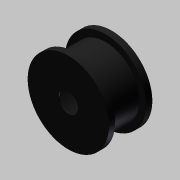
# Autodesk Inventor part: MSK01-06
Saved by Autodesk Inventor 2013 (Build 170138000, 138)
## iProperties
Created: 2011-08-17
Part Number: MSK01-06
Material: Nylon-6/6
Document SubType Name: Modeling
Designer: ERF
Mass: 1.99687 g
Surface Area: 10.0727 cm^2
Volume: 1.76715 cm^3
Density: 1.13 g/cm^3
Description: Smooth Idler Wheel
Stock Number: B17023
Vendor: buildlog.net
Author: ERF
Title: Smooth Idler Drum
Autodesk Inventor part; units mm, degrees
ref_plane "YZ Plane" through (0, 0, 0) normal (1, 0, 0) x (0, 1, 0)
ref_plane "XZ Plane" through (0, 0, 0) normal (0, 1, 0) x (-1, 0, 0)
ref_plane "XY Plane" through (0, 0, 0) normal (0, 0, 1) x (1, 0, 0)
sketch "Sketch1" plane through (0, 0, 0) normal (0, 0, 1) x (1, 0, 0)
  circle A0 centre (0, 0) radius 8.75
  circle A1 centre (0, 0) radius 2.5
  dimension "d0" = 17.5
  dimension "d1" = 5
  constraints: 2 centre point, 1 coincident
  measures "d0" diameter of A0
  measures "d1" diameter of A1
extrude "Extrusion1" add sketch "Sketch1" along normal blind 8
sketch "Sketch2" plane through (0, 0, 8) normal (0, 0, 1) x (1, 0, 0)
  circle A0 centre (0, 0) radius 2.5 projected
  circle A1 centre (0, 0) radius 8.75 projected
  circle A2 centre (0, 0) radius 10.5
  dimension "d4" = 21
  constraints: 1 centre point, 1 coincident
  measures "d4" diameter of A2
extrude "Extrusion2" add sketch "Sketch2" along normal blind 1.6 contours A1 | A2
sketch "Sketch3" plane through (0, 0, 0) normal (0, 0, -1) x (-1, 0, 0)
  circle A0 centre (0, 0) radius 2.5 projected
  circle A1 centre (0, 0) radius 8.75 projected
  circle A2 centre (0, 0) radius 10.5
  dimension "d7" = 21
  constraints: 1 centre point, 1 coincident
  measures "d7" diameter of A2
extrude "Extrusion3" add sketch "Sketch3" along normal blind 1.6 contours A1 | A2
sketch "Sketch5" plane through (0, 0, -1.6) normal (0, 0, -1) x (-1, 0, 0)
  circle A0 centre (0, 0) radius 2.5 projected
  circle A1 centre (0, 0) radius 10.5 projected
  circle A2 centre (0, 0) radius 8
  dimension "d11" = 16
  constraints: 1 centre point, 1 coincident
  measures "d11" diameter of A2
extrude "Extrusion4" cut sketch "Sketch5" against normal blind 11 contours A2
body "Solid1"
